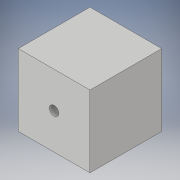
# Autodesk Inventor part: Motor test mount
Saved by Autodesk Inventor 2019 (Build 230136000, 136)
## iProperties
Created: 2020-03-18
Part Number: Motor test mount
Material: Generic
Document SubType Name: Modeling
Designer: 18186
Density: 1 g/cm^3
Appearance: Default
Author: 18186
Autodesk Inventor part; units mm, degrees
ref_plane "YZ Plane" through (0, 0, 0) normal (1, 0, 0) x (0, 1, 0)
ref_plane "XZ Plane" through (0, 0, 0) normal (0, 1, 0) x (-1, 0, 0)
ref_plane "XY Plane" through (0, 0, 0) normal (0, 0, 1) x (1, 0, 0)
sketch "Sketch1" plane through (0, 0, 0) normal (0, 0, 1) x (1, 0, 0)
  line L0 (-7.476, 7.4977) -> (17.924, 7.4977)
  line L1 (17.924, 7.4977) -> (17.924, -17.9023)
  line L2 (17.924, -17.9023) -> (-7.476, -17.9023)
  line L3 (-7.476, -17.9023) -> (-7.476, 7.4977)
  point P0 (0, 0)
  dimension "d0" = 25.4
  dimension "d1" = 25.4
  constraints: 8 end point, 2 parallel, 1 horizontal, 1 perpendicular
  measures "d0" distance of L1.end L2.end
  measures "d1" distance of L0.end L1.end
extrude "Extrusion1" add sketch "Sketch1" along normal blind 25.4
sketch "Sketch2" plane through (0, 0, 25.4) normal (0, 0, 1) x (1, 0, 0)
  line L0 (17.924, 7.4977) -> (-7.476, 7.4977) projected
  line L1 (-7.476, -17.9023) -> (17.924, -17.9023) projected
  line L2 (-7.476, 7.4977) -> (17.924, -17.9023) construction
  line L3 (-7.476, 7.4977) -> (-7.476, -17.9023) projected
  line L4 (17.924, 7.4977) -> (-7.476, -17.9023) construction
  circle A0 centre (5.224, -5.2023) radius 1.65
  point P0 (0, 0)
  dimension "d4" = 3.3
  constraints: 4 end point, 1 centre point, 1 midpoint
  measures "d4" diameter of A0
extrude "Extrusion2" cut sketch "Sketch2" against normal blind 5
body "Solid1"
